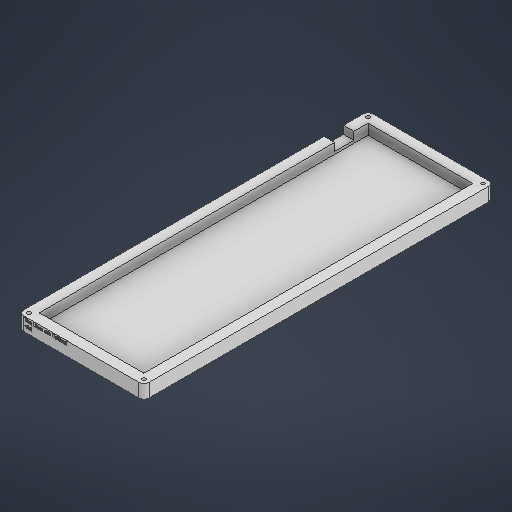
# Autodesk Inventor part: Bottom_Plate_MKey
Saved by Autodesk Inventor 2026 (Build 300175050, 175E)
## iProperties
Created: 2025-06-24
Part Number: Bottom_Plate_MKey
Material: Generic
Document SubType Name: Modeling
Designer: SaiAn
Density: 1 g/cm^3
Appearance: Default
Author: SaiAn
Autodesk Inventor part; units mm, degrees
ref_plane "YZ Plane" through (0, 0, 0) normal (1, 0, 0) x (0, 1, 0)
ref_plane "XZ Plane" through (0, 0, 0) normal (0, 1, 0) x (-1, 0, 0)
ref_plane "XY Plane" through (0, 0, 0) normal (0, 0, 1) x (1, 0, 0)
sketch "Sketch1" plane through (0, 0, 0) normal (0, 1, 0) x (-1, 0, 0)
  line L0 (0, 0) -> (100.47, 0)
  line L1 (100.47, 0) -> (100.47, -315.78)
  line L2 (100.47, -315.78) -> (0, -315.78)
  line L3 (0, -315.78) -> (0, 0)
  line L4 (110.47, 10) -> (-10, 10)
  line L5 (-10, 10) -> (-10, -325.78)
  line L6 (-10, -325.78) -> (110.47, -325.78)
  line L7 (110.47, -325.78) -> (110.47, 10)
  circle A0 centre (105.47, 5) radius 1.7
  circle A1 centre (-5, 5) radius 1.7
  circle A2 centre (-5, -320.78) radius 1.7
  circle A3 centre (105.47, -320.78) radius 1.7
  circle A4 centre (105.47, 5) radius 3
  circle A5 centre (-5, 5) radius 3
  circle A6 centre (-5, -320.78) radius 3
  circle A7 centre (105.47, -320.78) radius 3
  dimension "d0" = 100.47
  dimension "d1" = 315.78
  dimension "d2" = 120.47
  dimension "d3" = 335.78
  dimension "d4" = 10
  dimension "d5" = 10
  dimension "d6" = 3.4
  dimension "d7" = 3.4
  dimension "d8" = 3.4
  dimension "d9" = 3.4
  dimension "d10" = 5
  dimension "d11" = 5
  dimension "d12" = 5
  dimension "d13" = 5
  dimension "d14" = 5
  dimension "d15" = 5
  dimension "d16" = 5
  dimension "d17" = 5
  dimension "d18" = 6
  dimension "d19" = 6
  dimension "d20" = 6
  dimension "d21" = 6
  constraints: 16 end point, 8 centre point, 4 coincident, 4 parallel, 2 horizontal, 2 perpendicular
  measures "d0" distance of L1.end L2.end
  measures "d1" distance of L0.end L1.end
  measures "d2" distance of L6.end L5.end
  measures "d3" distance of L5.end L4.end
  measures "d4" distance between parallel lines of L1 L7
  measures "d5" distance between parallel lines of L6 L2
  measures "d6" diameter of A0
  measures "d7" diameter of A1
  measures "d8" diameter of A2
  measures "d9" diameter of A3
  measures "d10" distance from line of L7 A0.centre
  measures "d11" distance from line of L4 A0.centre
  measures "d12" distance from line of L5 A1.centre
  measures "d13" distance from line of L4 A1.centre
  measures "d14" distance from line of L5 A2.centre
  measures "d15" distance from line of L6 A2.centre
  measures "d16" distance from line of L7 A3.centre
  measures "d17" distance from line of L6 A3.centre
  measures "d18" diameter of A4
  measures "d19" diameter of A5
  measures "d20" diameter of A6
  measures "d21" diameter of A7
extrude "Extrusion1" add sketch "Sketch1" along normal blind 13 contours A4 | A5 | A6 | A7
extrude "Extrusion2" cut sketch "Sketch1" along normal blind 3.1 contours A4 | A5 | A6 | A7
extrude "Extrusion3" add sketch "Sketch1" along normal blind 13 contours L7 L6 L5 L4
extrude "Extrusion4" add sketch "Sketch1" along normal blind 3 contours L0 L1 L2 L3
sketch "Sketch3" plane through (0, 13, 0) normal (0, 1, 0) x (1, 0, 0)
  line L0 (-100.47, 0) -> (-100.47, 315.78) projected
  line L1 (-110.47, 325.78) -> (-110.47, -10) projected
  line L2 (-100.47, 302.18) -> (-110.47, 302.18)
  line L3 (-110.47, 302.18) -> (-110.47, 283.68)
  line L4 (-110.47, 283.68) -> (-100.47, 283.68)
  line L5 (-100.47, 283.68) -> (-100.47, 302.18)
  line L6 (10, 325.78) -> (-110.47, 325.78) projected
  point P0 (0, 0)
  dimension "d30" = 18.5
  dimension "d31" = 23.6
  constraints: 8 end point, 2 parallel, 2 point on line, 1 horizontal, 1 perpendicular
  measures "d30" distance of L3.end L2.end
  measures "d31" distance between parallel lines of L6 L2
extrude "Extrusion5" cut sketch "Sketch3" against normal blind 7.5
fillet "Fillet1" radius 5 3 edges at (-110.47, 6.5, -325.78) (10, 6.5, -325.78) (10, 6.5, 10)
fillet "Fillet2" radius 5 1 edges at (-110.47, 6.5, 10)
sketch "Sketch6" plane through (5, 0, 10) normal (0, 0, 1) x (1, 0, 0)
  line L0 (-109.6775, 12.2392) -> (-5.1074, 12.2392) construction
  line L1 (-5.1074, 12.2392) -> (-5.1074, 1.2883) construction
  line L2 (-5.1074, 1.2883) -> (-109.6775, 1.2883) construction
  line L3 (-109.6775, 1.2883) -> (-109.6775, 12.2392) construction
  line L4 (-108.6574, 9.0554) -> (-108.6574, 11.7427)
  line L5 (-108.6574, 11.7427) -> (-109.68, 11.7427)
  line L6 (-109.68, 11.7427) -> (-109.68, 12.1034)
  line L7 (-109.68, 12.1034) -> (-107.2297, 12.1034)
  line L8 (-107.2297, 12.1034) -> (-107.2297, 11.7427)
  line L9 (-107.2297, 11.7427) -> (-108.2523, 11.7427)
  line L10 (-108.2523, 11.7427) -> (-108.2523, 9.0554)
  line L11 (-108.2523, 9.0554) -> (-108.6574, 9.0554)
  line L12 (-105.1549, 9.0554) -> (-105.5402, 9.0554)
  line L13 (-105.5402, 9.0554) -> (-105.5402, 10.3595)
  spline S0 degree 2 poles (-105.5402, 10.3595) (-105.5402, 10.5176) (-105.5699, 10.7893) (-105.6143, 10.8708) knots 0 0 0 1 2 2 2
  spline S1 degree 2 poles (-105.6143, 10.8708) (-105.6612, 10.9573) (-105.8292, 11.0413) (-105.9725, 11.0413) knots 0 0 0 1 2 2 2
  spline S2 degree 2 poles (-105.9725, 11.0413) (-106.1157, 11.0413) (-106.4195, 10.8881) (-106.5653, 10.7646) knots 0 0 0 1 2 2 2
  line L14 (-106.5653, 10.7646) -> (-106.5653, 9.0554)
  line L15 (-106.5653, 9.0554) -> (-106.9506, 9.0554)
  line L16 (-106.9506, 9.0554) -> (-106.9506, 12.2392)
  line L17 (-106.9506, 12.2392) -> (-106.5653, 12.2392)
  line L18 (-106.5653, 12.2392) -> (-106.5653, 11.0882)
  spline S3 degree 2 poles (-106.5653, 11.0882) (-106.3924, 11.2438) (-106.0589, 11.4068) (-105.8712, 11.4068) knots 0 0 0 1 2 2 2
  spline S4 degree 2 poles (-105.8712, 11.4068) (-105.5353, 11.4068) (-105.1549, 10.9622) (-105.1549, 10.5398) knots 0 0 0 1 2 2 2
  line L19 (-105.1549, 10.5398) -> (-105.1549, 9.0554)
  spline S5 degree 2 poles (-103.621, 9.0035) (-104.1694, 9.0035) (-104.772, 9.6185) (-104.772, 10.1866) knots 0 0 0 1 2 2 2
  spline S6 degree 2 poles (-104.772, 10.1866) (-104.772, 10.7449) (-104.1867, 11.4068) (-103.7149, 11.4068) knots 0 0 0 1 2 2 2
  spline S7 degree 2 poles (-103.7149, 11.4068) (-103.5025, 11.4068) (-103.1739, 11.2833) (-103.0529, 11.1524) knots 0 0 0 1 2 2 2
  spline S8 degree 2 poles (-103.0529, 11.1524) (-102.9294, 11.0215) (-102.7985, 10.6436) (-102.7985, 10.3694) knots 0 0 0 1 2 2 2
  line L20 (-102.7985, 10.3694) -> (-102.7985, 10.1595)
  line L21 (-102.7985, 10.1595) -> (-104.3818, 10.1595)
  spline S9 degree 2 poles (-104.3818, 10.1595) (-104.3818, 9.7618) (-103.9816, 9.3394) (-103.626, 9.3394) knots 0 0 0 1 2 2 2
  spline S10 degree 2 poles (-103.626, 9.3394) (-103.5, 9.3394) (-103.2555, 9.3962) (-103.1567, 9.4407) knots 0 0 0 1 2 2 2
  spline S11 degree 2 poles (-103.1567, 9.4407) (-103.0529, 9.4901) (-102.9097, 9.5765) (-102.8627, 9.6161) knots 0 0 0 1 2 2 2
  line L22 (-102.8627, 9.6161) -> (-102.8405, 9.6161)
  line L23 (-102.8405, 9.6161) -> (-102.8405, 9.1962)
  spline S12 degree 2 poles (-102.8405, 9.1962) (-102.9072, 9.169) (-103.1097, 9.0899) (-103.1888, 9.0677) knots 0 0 0 1 2 2 2
  spline S13 degree 2 poles (-103.1888, 9.0677) (-103.2999, 9.0356) (-103.4827, 9.0035) (-103.621, 9.0035) knots 0 0 0 1 2 2 2
  spline S14 degree 2 poles (-103.1739, 10.4534) (-103.1789, 10.609) (-103.2431, 10.8362) (-103.3049, 10.9128) knots 0 0 0 1 2 2 2
  spline S15 degree 2 poles (-103.3049, 10.9128) (-103.3715, 10.9993) (-103.5815, 11.0907) (-103.7371, 11.0907) knots 0 0 0 1 2 2 2
  spline S16 degree 2 poles (-103.7371, 11.0907) (-103.8902, 11.0907) (-104.1051, 10.9993) (-104.1941, 10.9103) knots 0 0 0 1 2 2 2
  spline S17 degree 2 poles (-104.1941, 10.9103) (-104.2805, 10.819) (-104.3694, 10.5991) (-104.3818, 10.4534) knots 0 0 0 1 2 2 2
  line L24 (-104.3818, 10.4534) -> (-103.1739, 10.4534)
  line L25 (-99.3034, 9.0554) -> (-101.0695, 9.0554)
  line L26 (-101.0695, 9.0554) -> (-101.0695, 12.1034)
  line L27 (-101.0695, 12.1034) -> (-100.6644, 12.1034)
  line L28 (-100.6644, 12.1034) -> (-100.6644, 9.416)
  line L29 (-100.6644, 9.416) -> (-99.3034, 9.416)
  line L30 (-99.3034, 9.416) -> (-99.3034, 9.0554)
  line L31 (-98.6217, 9.0554) -> (-99.007, 9.0554)
  line L32 (-99.007, 9.0554) -> (-99.007, 11.3426)
  line L33 (-99.007, 11.3426) -> (-98.6217, 11.3426)
  line L34 (-98.6217, 11.3426) -> (-98.6217, 9.0554)
  line L35 (-98.5945, 11.723) -> (-99.0317, 11.723)
  line L36 (-99.0317, 11.723) -> (-99.0317, 12.1231)
  line L37 (-99.0317, 12.1231) -> (-98.5945, 12.1231)
  line L38 (-98.5945, 12.1231) -> (-98.5945, 11.723)
  line L39 (-96.2604, 9.0554) -> (-96.6457, 9.0554)
  line L40 (-96.6457, 9.0554) -> (-96.6457, 10.3595)
  spline S18 degree 2 poles (-96.6457, 10.3595) (-96.6457, 10.5176) (-96.6753, 10.7893) (-96.7198, 10.8708) knots 0 0 0 1 2 2 2
  spline S19 degree 2 poles (-96.7198, 10.8708) (-96.7667, 10.9573) (-96.9347, 11.0413) (-97.0779, 11.0413) knots 0 0 0 1 2 2 2
  spline S20 degree 2 poles (-97.0779, 11.0413) (-97.2212, 11.0413) (-97.525, 10.8881) (-97.6707, 10.7646) knots 0 0 0 1 2 2 2
  line L41 (-97.6707, 10.7646) -> (-97.6707, 9.0554)
  line L42 (-97.6707, 9.0554) -> (-98.0561, 9.0554)
  line L43 (-98.0561, 9.0554) -> (-98.0561, 11.3426)
  line L44 (-98.0561, 11.3426) -> (-97.6707, 11.3426)
  line L45 (-97.6707, 11.3426) -> (-97.6707, 11.0882)
  spline S21 degree 2 poles (-97.6707, 11.0882) (-97.4978, 11.2438) (-97.1644, 11.4068) (-96.9767, 11.4068) knots 0 0 0 1 2 2 2
  spline S22 degree 2 poles (-96.9767, 11.4068) (-96.6408, 11.4068) (-96.2604, 10.9622) (-96.2604, 10.5398) knots 0 0 0 1 2 2 2
  line L46 (-96.2604, 10.5398) -> (-96.2604, 9.0554)
  spline S23 degree 2 poles (-94.7265, 9.0035) (-95.2748, 9.0035) (-95.8775, 9.6185) (-95.8775, 10.1866) knots 0 0 0 1 2 2 2
  spline S24 degree 2 poles (-95.8775, 10.1866) (-95.8775, 10.7449) (-95.2921, 11.4068) (-94.8203, 11.4068) knots 0 0 0 1 2 2 2
  spline S25 degree 2 poles (-94.8203, 11.4068) (-94.6079, 11.4068) (-94.2794, 11.2833) (-94.1584, 11.1524) knots 0 0 0 1 2 2 2
  spline S26 degree 2 poles (-94.1584, 11.1524) (-94.0349, 11.0215) (-93.904, 10.6436) (-93.904, 10.3694) knots 0 0 0 1 2 2 2
  line L47 (-93.904, 10.3694) -> (-93.904, 10.1595)
  line L48 (-93.904, 10.1595) -> (-95.4873, 10.1595)
  spline S27 degree 2 poles (-95.4873, 10.1595) (-95.4873, 9.7618) (-95.0871, 9.3394) (-94.7314, 9.3394) knots 0 0 0 1 2 2 2
  spline S28 degree 2 poles (-94.7314, 9.3394) (-94.6055, 9.3394) (-94.3609, 9.3962) (-94.2621, 9.4407) knots 0 0 0 1 2 2 2
  spline S29 degree 2 poles (-94.2621, 9.4407) (-94.1584, 9.4901) (-94.0151, 9.5765) (-93.9682, 9.6161) knots 0 0 0 1 2 2 2
  line L49 (-93.9682, 9.6161) -> (-93.946, 9.6161)
  line L50 (-93.946, 9.6161) -> (-93.946, 9.1962)
  spline S30 degree 2 poles (-93.946, 9.1962) (-94.0127, 9.169) (-94.2152, 9.0899) (-94.2942, 9.0677) knots 0 0 0 1 2 2 2
  spline S31 degree 2 poles (-94.2942, 9.0677) (-94.4054, 9.0356) (-94.5882, 9.0035) (-94.7265, 9.0035) knots 0 0 0 1 2 2 2
  spline S32 degree 2 poles (-94.2794, 10.4534) (-94.2844, 10.609) (-94.3486, 10.8362) (-94.4103, 10.9128) knots 0 0 0 1 2 2 2
  spline S33 degree 2 poles (-94.4103, 10.9128) (-94.477, 10.9993) (-94.687, 11.0907) (-94.8426, 11.0907) knots 0 0 0 1 2 2 2
  spline S34 degree 2 poles (-94.8426, 11.0907) (-94.9957, 11.0907) (-95.2106, 10.9993) (-95.2995, 10.9103) knots 0 0 0 1 2 2 2
  spline S35 degree 2 poles (-95.2995, 10.9103) (-95.386, 10.819) (-95.4749, 10.5991) (-95.4873, 10.4534) knots 0 0 0 1 2 2 2
  line L51 (-95.4873, 10.4534) -> (-94.2794, 10.4534)
  spline S36 degree 2 poles (-92.8962, 9.001) (-93.1259, 9.001) (-93.5236, 9.1245) (-93.6545, 9.1937) knots 0 0 0 1 2 2 2
  line L52 (-93.6545, 9.1937) -> (-93.6545, 9.6259)
  line L53 (-93.6545, 9.6259) -> (-93.6347, 9.6259)
  spline S37 degree 2 poles (-93.6347, 9.6259) (-93.5853, 9.5864) (-93.452, 9.4926) (-93.3408, 9.4407) knots 0 0 0 1 2 2 2
  spline S38 degree 2 poles (-93.3408, 9.4407) (-93.2445, 9.3938) (-93.0074, 9.3246) (-92.8814, 9.3246) knots 0 0 0 1 2 2 2
  spline S39 degree 2 poles (-92.8814, 9.3246) (-92.79, 9.3246) (-92.58, 9.3666) (-92.5306, 9.4012) knots 0 0 0 1 2 2 2
  spline S40 degree 2 poles (-92.5306, 9.4012) (-92.459, 9.4481) (-92.3948, 9.5543) (-92.3948, 9.663) knots 0 0 0 1 2 2 2
  spline S41 degree 2 poles (-92.3948, 9.663) (-92.3948, 9.7988) (-92.543, 9.9396) (-92.7332, 9.9866) knots 0 0 0 1 2 2 2
  spline S42 degree 2 poles (-92.7332, 9.9866) (-92.8073, 10.0039) (-93.0444, 10.0533) (-93.1457, 10.0804) knots 0 0 0 1 2 2 2
  spline S43 degree 2 poles (-93.1457, 10.0804) (-93.4075, 10.157) (-93.6446, 10.4732) (-93.6446, 10.6979) knots 0 0 0 1 2 2 2
  spline S44 degree 2 poles (-93.6446, 10.6979) (-93.6446, 11.0091) (-93.1778, 11.3969) (-92.7925, 11.3969) knots 0 0 0 1 2 2 2
  spline S45 degree 2 poles (-92.7925, 11.3969) (-92.6023, 11.3969) (-92.217, 11.3031) (-92.086, 11.2314) knots 0 0 0 1 2 2 2
  line L54 (-92.086, 11.2314) -> (-92.086, 10.819)
  line L55 (-92.086, 10.819) -> (-92.1058, 10.819)
  spline S46 degree 2 poles (-92.1058, 10.819) (-92.254, 10.9375) (-92.6146, 11.0734) (-92.7999, 11.0734) knots 0 0 0 1 2 2 2
  spline S47 degree 2 poles (-92.7999, 11.0734) (-92.9901, 11.0734) (-93.2519, 10.9128) (-93.2519, 10.7523) knots 0 0 0 1 2 2 2
  spline S48 degree 2 poles (-93.2519, 10.7523) (-93.2519, 10.6065) (-93.0963, 10.4657) (-92.9234, 10.4213) knots 0 0 0 1 2 2 2
  spline S49 degree 2 poles (-92.9234, 10.4213) (-92.8394, 10.3991) (-92.627, 10.3546) (-92.5109, 10.3274) knots 0 0 0 1 2 2 2
  spline S50 degree 2 poles (-92.5109, 10.3274) (-92.2589, 10.2632) (-92.0021, 9.9693) (-92.0021, 9.7149) knots 0 0 0 1 2 2 2
  spline S51 degree 2 poles (-92.0021, 9.7149) (-92.0021, 9.5667) (-92.1182, 9.3048) (-92.2318, 9.2085) knots 0 0 0 1 2 2 2
  spline S52 degree 2 poles (-92.2318, 9.2085) (-92.3528, 9.1072) (-92.6616, 9.001) (-92.8962, 9.001) knots 0 0 0 1 2 2 2
  spline S53 degree 2 poles (-89.0603, 9.2974) (-89.1072, 9.2628) (-89.2653, 9.1393) (-89.3394, 9.1023) knots 0 0 0 1 2 2 2
  spline S54 degree 2 poles (-89.3394, 9.1023) (-89.4407, 9.048) (-89.6308, 8.9911) (-89.8037, 8.9911) knots 0 0 0 1 2 2 2
  spline S55 degree 2 poles (-89.8037, 8.9911) (-89.9445, 8.9911) (-90.1989, 9.0974) (-90.2953, 9.1937) knots 0 0 0 1 2 2 2
  spline S56 degree 2 poles (-90.2953, 9.1937) (-90.3867, 9.2875) (-90.4978, 9.5642) (-90.4978, 9.7173) knots 0 0 0 1 2 2 2
  spline S57 degree 2 poles (-90.4978, 9.7173) (-90.4978, 9.9544) (-90.2977, 10.2904) (-90.0804, 10.3867) knots 0 0 0 1 2 2 2
  spline S58 degree 2 poles (-90.0804, 10.3867) (-89.8877, 10.4756) (-89.3641, 10.5423) (-89.0603, 10.5596) knots 0 0 0 1 2 2 2
  line L56 (-89.0603, 10.5596) -> (-89.0603, 10.6337)
  spline S59 degree 2 poles (-89.0603, 10.6337) (-89.0603, 10.7671) (-89.1418, 10.9326) (-89.2159, 10.9795) knots 0 0 0 1 2 2 2
  spline S60 degree 2 poles (-89.2159, 10.9795) (-89.29, 11.0264) (-89.5024, 11.0561) (-89.616, 11.0561) knots 0 0 0 1 2 2 2
  spline S61 degree 2 poles (-89.616, 11.0561) (-89.7494, 11.0561) (-90.11, 10.977) (-90.2903, 10.9005) knots 0 0 0 1 2 2 2
  line L57 (-90.2903, 10.9005) -> (-90.3126, 10.9005)
  line L58 (-90.3126, 10.9005) -> (-90.3126, 11.2932)
  spline S62 degree 2 poles (-90.3126, 11.2932) (-90.2064, 11.3228) (-89.8087, 11.3969) (-89.6136, 11.3969) knots 0 0 0 1 2 2 2
  spline S63 degree 2 poles (-89.6136, 11.3969) (-89.3764, 11.3969) (-89.0529, 11.3228) (-88.9244, 11.2265) knots 0 0 0 1 2 2 2
  spline S64 degree 2 poles (-88.9244, 11.2265) (-88.7984, 11.1326) (-88.6749, 10.8338) (-88.6749, 10.6189) knots 0 0 0 1 2 2 2
  line L59 (-88.6749, 10.6189) -> (-88.6749, 9.0554)
  line L60 (-88.6749, 9.0554) -> (-89.0603, 9.0554)
  line L61 (-89.0603, 9.0554) -> (-89.0603, 9.2974)
  line L62 (-89.0603, 9.6185) -> (-89.0603, 10.2533)
  spline S65 degree 2 poles (-89.0603, 10.2533) (-89.1986, 10.241) (-89.616, 10.199) (-89.7469, 10.1595) knots 0 0 0 1 2 2 2
  spline S66 degree 2 poles (-89.7469, 10.1595) (-89.9001, 10.1125) (-90.1001, 9.9174) (-90.1001, 9.7445) knots 0 0 0 1 2 2 2
  spline S67 degree 2 poles (-90.1001, 9.7445) (-90.1001, 9.5469) (-89.8778, 9.3468) (-89.6654, 9.3468) knots 0 0 0 1 2 2 2
  spline S68 degree 2 poles (-89.6654, 9.3468) (-89.4851, 9.3468) (-89.1887, 9.5024) (-89.0603, 9.6185) knots 0 0 0 1 2 2 2
  line L63 (-86.9212, 10.9301) -> (-86.941, 10.9301)
  spline S69 degree 2 poles (-86.941, 10.9301) (-86.9855, 10.9425) (-87.0818, 10.9474) (-87.1485, 10.9474) knots 0 0 0 1 2 2 2
  spline S70 degree 2 poles (-87.1485, 10.9474) (-87.3041, 10.9474) (-87.6104, 10.8115) (-87.7487, 10.6782) knots 0 0 0 1 2 2 2
  line L64 (-87.7487, 10.6782) -> (-87.7487, 9.0554)
  line L65 (-87.7487, 9.0554) -> (-88.134, 9.0554)
  line L66 (-88.134, 9.0554) -> (-88.134, 11.3426)
  line L67 (-88.134, 11.3426) -> (-87.7487, 11.3426)
  line L68 (-87.7487, 11.3426) -> (-87.7487, 11.0017)
  spline S71 degree 2 poles (-87.7487, 11.0017) (-87.5387, 11.1895) (-87.225, 11.3426) (-87.0768, 11.3426) knots 0 0 0 1 2 2 2
  spline S72 degree 2 poles (-87.0768, 11.3426) (-87.0176, 11.3426) (-86.9583, 11.3377) (-86.9212, 11.3302) knots 0 0 0 1 2 2 2
  line L69 (-86.9212, 11.3302) -> (-86.9212, 10.9301)
  spline S73 degree 2 poles (-85.6294, 9.0035) (-86.1778, 9.0035) (-86.7804, 9.6185) (-86.7804, 10.1866) knots 0 0 0 1 2 2 2
  spline S74 degree 2 poles (-86.7804, 10.1866) (-86.7804, 10.7449) (-86.1951, 11.4068) (-85.7233, 11.4068) knots 0 0 0 1 2 2 2
  spline S75 degree 2 poles (-85.7233, 11.4068) (-85.5109, 11.4068) (-85.1823, 11.2833) (-85.0613, 11.1524) knots 0 0 0 1 2 2 2
  spline S76 degree 2 poles (-85.0613, 11.1524) (-84.9378, 11.0215) (-84.8069, 10.6436) (-84.8069, 10.3694) knots 0 0 0 1 2 2 2
  line L70 (-84.8069, 10.3694) -> (-84.8069, 10.1595)
  line L71 (-84.8069, 10.1595) -> (-86.3902, 10.1595)
  spline S77 degree 2 poles (-86.3902, 10.1595) (-86.3902, 9.7618) (-85.99, 9.3394) (-85.6344, 9.3394) knots 0 0 0 1 2 2 2
  spline S78 degree 2 poles (-85.6344, 9.3394) (-85.5084, 9.3394) (-85.2639, 9.3962) (-85.1651, 9.4407) knots 0 0 0 1 2 2 2
  spline S79 degree 2 poles (-85.1651, 9.4407) (-85.0613, 9.4901) (-84.9181, 9.5765) (-84.8711, 9.6161) knots 0 0 0 1 2 2 2
  line L72 (-84.8711, 9.6161) -> (-84.8489, 9.6161)
  line L73 (-84.8489, 9.6161) -> (-84.8489, 9.1962)
  spline S80 degree 2 poles (-84.8489, 9.1962) (-84.9156, 9.169) (-85.1181, 9.0899) (-85.1972, 9.0677) knots 0 0 0 1 2 2 2
  spline S81 degree 2 poles (-85.1972, 9.0677) (-85.3083, 9.0356) (-85.4911, 9.0035) (-85.6294, 9.0035) knots 0 0 0 1 2 2 2
  spline S82 degree 2 poles (-85.1823, 10.4534) (-85.1873, 10.609) (-85.2515, 10.8362) (-85.3133, 10.9128) knots 0 0 0 1 2 2 2
  spline S83 degree 2 poles (-85.3133, 10.9128) (-85.3799, 10.9993) (-85.5899, 11.0907) (-85.7455, 11.0907) knots 0 0 0 1 2 2 2
  spline S84 degree 2 poles (-85.7455, 11.0907) (-85.8986, 11.0907) (-86.1135, 10.9993) (-86.2025, 10.9103) knots 0 0 0 1 2 2 2
  spline S85 degree 2 poles (-86.2025, 10.9103) (-86.2889, 10.819) (-86.3778, 10.5991) (-86.3902, 10.4534) knots 0 0 0 1 2 2 2
  line L74 (-86.3902, 10.4534) -> (-85.1823, 10.4534)
  spline S86 degree 2 poles (-80.9216, 11.7551) (-80.7487, 11.5526) (-80.556, 10.9597) (-80.556, 10.5794) knots 0 0 0 1 2 2 2
  spline S87 degree 2 poles (-80.556, 10.5794) (-80.556, 10.2089) (-80.7437, 9.6086) (-80.9216, 9.4061) knots 0 0 0 1 2 2 2
  spline S88 degree 2 poles (-80.9216, 9.4061) (-81.1093, 9.1937) (-81.6058, 8.9911) (-81.9046, 8.9911) knots 0 0 0 1 2 2 2
  spline S89 degree 2 poles (-81.9046, 8.9911) (-82.2134, 8.9911) (-82.7074, 9.2011) (-82.8877, 9.4061) knots 0 0 0 1 2 2 2
  spline S90 degree 2 poles (-82.8877, 9.4061) (-83.0631, 9.6086) (-83.2508, 10.2039) (-83.2508, 10.5794) knots 0 0 0 1 2 2 2
  spline S91 degree 2 poles (-83.2508, 10.5794) (-83.2508, 10.9622) (-83.0606, 11.5451) (-82.8852, 11.7551) knots 0 0 0 1 2 2 2
  spline S92 degree 2 poles (-82.8852, 11.7551) (-82.7074, 11.9576) (-82.2109, 12.1676) (-81.9046, 12.1676) knots 0 0 0 1 2 2 2
  spline S93 degree 2 poles (-81.9046, 12.1676) (-81.5934, 12.1676) (-81.0945, 11.9502) (-80.9216, 11.7551) knots 0 0 0 1 2 2 2
  spline S94 degree 2 poles (-80.9784, 10.5794) (-80.9784, 10.8807) (-81.1093, 11.3475) (-81.2278, 11.5007) knots 0 0 0 1 2 2 2
  spline S95 degree 2 poles (-81.2278, 11.5007) (-81.3489, 11.6588) (-81.6897, 11.8168) (-81.9022, 11.8168) knots 0 0 0 1 2 2 2
  spline S96 degree 2 poles (-81.9022, 11.8168) (-82.122, 11.8168) (-82.453, 11.6637) (-82.5789, 11.5007) knots 0 0 0 1 2 2 2
  spline S97 degree 2 poles (-82.5789, 11.5007) (-82.7, 11.3451) (-82.8284, 10.8758) (-82.8284, 10.5794) knots 0 0 0 1 2 2 2
  spline S98 degree 2 poles (-82.8284, 10.5794) (-82.8284, 9.9791) (-82.3245, 9.3419) (-81.9022, 9.3419) knots 0 0 0 1 2 2 2
  spline S99 degree 2 poles (-81.9022, 9.3419) (-81.4798, 9.3419) (-80.9784, 9.9791) (-80.9784, 10.5794) knots 0 0 0 1 2 2 2
  spline S100 degree 2 poles (-78.2243, 10.2607) (-78.2243, 9.6877) (-78.7702, 9.0109) (-79.1876, 9.0109) knots 0 0 0 1 2 2 2
  spline S101 degree 2 poles (-79.1876, 9.0109) (-79.358, 9.0109) (-79.6199, 9.0899) (-79.7557, 9.1715) knots 0 0 0 1 2 2 2
  line L75 (-79.7557, 9.1715) -> (-79.7557, 8.2131)
  line L76 (-79.7557, 8.2131) -> (-80.141, 8.2131)
  line L77 (-80.141, 8.2131) -> (-80.141, 11.3426)
  line L78 (-80.141, 11.3426) -> (-79.7557, 11.3426)
  line L79 (-79.7557, 11.3426) -> (-79.7557, 11.103)
  spline S102 degree 2 poles (-79.7557, 11.103) (-79.6125, 11.2339) (-79.2617, 11.4068) (-79.0567, 11.4068) knots 0 0 0 1 2 2 2
  spline S103 degree 2 poles (-79.0567, 11.4068) (-78.664, 11.4068) (-78.2243, 10.7844) (-78.2243, 10.2607) knots 0 0 0 1 2 2 2
  spline S104 degree 2 poles (-78.622, 10.2163) (-78.622, 10.609) (-78.8715, 11.0413) (-79.1506, 11.0413) knots 0 0 0 1 2 2 2
  spline S105 degree 2 poles (-79.1506, 11.0413) (-79.3136, 11.0413) (-79.6199, 10.8955) (-79.7557, 10.7819) knots 0 0 0 1 2 2 2
  line L80 (-79.7557, 10.7819) -> (-79.7557, 9.4827)
  spline S106 degree 2 poles (-79.7557, 9.4827) (-79.605, 9.411) (-79.3902, 9.3567) (-79.2518, 9.3567) knots 0 0 0 1 2 2 2
  spline S107 degree 2 poles (-79.2518, 9.3567) (-78.953, 9.3567) (-78.622, 9.7964) (-78.622, 10.2163) knots 0 0 0 1 2 2 2
  spline S108 degree 2 poles (-77.1326, 9.0109) (-77.4463, 9.0109) (-77.7995, 9.3691) (-77.7995, 9.7568) knots 0 0 0 1 2 2 2
  line L81 (-77.7995, 9.7568) -> (-77.7995, 11.024)
  line L82 (-77.7995, 11.024) -> (-78.0588, 11.024)
  line L83 (-78.0588, 11.024) -> (-78.0588, 11.3426)
  line L84 (-78.0588, 11.3426) -> (-77.7995, 11.3426)
  line L85 (-77.7995, 11.3426) -> (-77.7995, 11.9996)
  line L86 (-77.7995, 11.9996) -> (-77.4141, 11.9996)
  line L87 (-77.4141, 11.9996) -> (-77.4141, 11.3426)
  line L88 (-77.4141, 11.3426) -> (-76.7052, 11.3426)
  line L89 (-76.7052, 11.3426) -> (-76.7052, 11.024)
  line L90 (-76.7052, 11.024) -> (-77.4141, 11.024)
  line L91 (-77.4141, 11.024) -> (-77.4141, 9.9347)
  spline S109 degree 2 poles (-77.4141, 9.9347) (-77.4141, 9.7618) (-77.4018, 9.5716) (-77.3598, 9.4901) knots 0 0 0 1 2 2 2
  spline S110 degree 2 poles (-77.3598, 9.4901) (-77.3252, 9.4185) (-77.1696, 9.3468) (-77.0362, 9.3468) knots 0 0 0 1 2 2 2
  spline S111 degree 2 poles (-77.0362, 9.3468) (-76.9424, 9.3468) (-76.767, 9.4036) (-76.7275, 9.4209) knots 0 0 0 1 2 2 2
  line L92 (-76.7275, 9.4209) -> (-76.7052, 9.4209)
  line L93 (-76.7052, 9.4209) -> (-76.7052, 9.0751)
  spline S112 degree 2 poles (-76.7052, 9.0751) (-76.8139, 9.0455) (-77.0362, 9.0109) (-77.1326, 9.0109) knots 0 0 0 1 2 2 2
  line L94 (-76.0285, 9.0554) -> (-76.4138, 9.0554)
  line L95 (-76.4138, 9.0554) -> (-76.4138, 11.3426)
  line L96 (-76.4138, 11.3426) -> (-76.0285, 11.3426)
  line L97 (-76.0285, 11.3426) -> (-76.0285, 9.0554)
  line L98 (-76.0013, 11.723) -> (-76.4385, 11.723)
  line L99 (-76.4385, 11.723) -> (-76.4385, 12.1231)
  line L100 (-76.4385, 12.1231) -> (-76.0013, 12.1231)
  line L101 (-76.0013, 12.1231) -> (-76.0013, 11.723)
  line L102 (-72.8693, 9.0554) -> (-72.8693, 10.3793)
  spline S113 degree 2 poles (-72.8693, 10.3793) (-72.8693, 10.5374) (-72.894, 10.8066) (-72.9335, 10.8807) knots 0 0 0 1 2 2 2
  spline S114 degree 2 poles (-72.9335, 10.8807) (-72.9731, 10.9622) (-73.1237, 11.0413) (-73.2546, 11.0413) knots 0 0 0 1 2 2 2
  spline S115 degree 2 poles (-73.2546, 11.0413) (-73.3732, 11.0413) (-73.6449, 10.8955) (-73.7882, 10.7572) knots 0 0 0 1 2 2 2
  spline S116 degree 2 poles (-73.7882, 10.7572) (-73.7857, 10.7226) (-73.7808, 10.6263) (-73.7808, 10.5621) knots 0 0 0 1 2 2 2
  line L103 (-73.7808, 10.5621) -> (-73.7808, 9.0554)
  line L104 (-73.7808, 9.0554) -> (-74.1661, 9.0554)
  line L105 (-74.1661, 9.0554) -> (-74.1661, 10.3793)
  spline S117 degree 2 poles (-74.1661, 10.3793) (-74.1661, 10.5374) (-74.1908, 10.8066) (-74.2303, 10.8807) knots 0 0 0 1 2 2 2
  spline S118 degree 2 poles (-74.2303, 10.8807) (-74.2698, 10.9622) (-74.4205, 11.0413) (-74.5514, 11.0413) knots 0 0 0 1 2 2 2
  spline S119 degree 2 poles (-74.5514, 11.0413) (-74.6749, 11.0413) (-74.9491, 10.8856) (-75.0775, 10.7646) knots 0 0 0 1 2 2 2
  line L106 (-75.0775, 10.7646) -> (-75.0775, 9.0554)
  line L107 (-75.0775, 9.0554) -> (-75.4628, 9.0554)
  line L108 (-75.4628, 9.0554) -> (-75.4628, 11.3426)
  line L109 (-75.4628, 11.3426) -> (-75.0775, 11.3426)
  line L110 (-75.0775, 11.3426) -> (-75.0775, 11.0907)
  spline S120 degree 2 poles (-75.0775, 11.0907) (-74.9268, 11.2413) (-74.6304, 11.4068) (-74.4526, 11.4068) knots 0 0 0 1 2 2 2
  spline S121 degree 2 poles (-74.4526, 11.4068) (-74.2501, 11.4068) (-73.9364, 11.2216) (-73.8549, 11.0116) knots 0 0 0 1 2 2 2
  spline S122 degree 2 poles (-73.8549, 11.0116) (-73.6795, 11.2067) (-73.3485, 11.4068) (-73.1558, 11.4068) knots 0 0 0 1 2 2 2
  spline S123 degree 2 poles (-73.1558, 11.4068) (-73.0076, 11.4068) (-72.7656, 11.3154) (-72.6767, 11.2117) knots 0 0 0 1 2 2 2
  spline S124 degree 2 poles (-72.6767, 11.2117) (-72.5853, 11.1079) (-72.484, 10.7967) (-72.484, 10.5621) knots 0 0 0 1 2 2 2
  line L111 (-72.484, 10.5621) -> (-72.484, 9.0554)
  line L112 (-72.484, 9.0554) -> (-72.8693, 9.0554)
  spline S125 degree 2 poles (-70.6685, 9.2974) (-70.7155, 9.2628) (-70.8735, 9.1393) (-70.9476, 9.1023) knots 0 0 0 1 2 2 2
  spline S126 degree 2 poles (-70.9476, 9.1023) (-71.0489, 9.048) (-71.2391, 8.9911) (-71.412, 8.9911) knots 0 0 0 1 2 2 2
  spline S127 degree 2 poles (-71.412, 8.9911) (-71.5528, 8.9911) (-71.8072, 9.0974) (-71.9035, 9.1937) knots 0 0 0 1 2 2 2
  spline S128 degree 2 poles (-71.9035, 9.1937) (-71.9949, 9.2875) (-72.1061, 9.5642) (-72.1061, 9.7173) knots 0 0 0 1 2 2 2
  spline S129 degree 2 poles (-72.1061, 9.7173) (-72.1061, 9.9544) (-71.906, 10.2904) (-71.6886, 10.3867) knots 0 0 0 1 2 2 2
  spline S130 degree 2 poles (-71.6886, 10.3867) (-71.496, 10.4756) (-70.9723, 10.5423) (-70.6685, 10.5596) knots 0 0 0 1 2 2 2
  line L113 (-70.6685, 10.5596) -> (-70.6685, 10.6337)
  spline S131 degree 2 poles (-70.6685, 10.6337) (-70.6685, 10.7671) (-70.75, 10.9326) (-70.8241, 10.9795) knots 0 0 0 1 2 2 2
  spline S132 degree 2 poles (-70.8241, 10.9795) (-70.8982, 11.0264) (-71.1107, 11.0561) (-71.2243, 11.0561) knots 0 0 0 1 2 2 2
  spline S133 degree 2 poles (-71.2243, 11.0561) (-71.3577, 11.0561) (-71.7183, 10.977) (-71.8986, 10.9005) knots 0 0 0 1 2 2 2
  line L114 (-71.8986, 10.9005) -> (-71.9208, 10.9005)
  line L115 (-71.9208, 10.9005) -> (-71.9208, 11.2932)
  spline S134 degree 2 poles (-71.9208, 11.2932) (-71.8146, 11.3228) (-71.4169, 11.3969) (-71.2218, 11.3969) knots 0 0 0 1 2 2 2
  spline S135 degree 2 poles (-71.2218, 11.3969) (-70.9847, 11.3969) (-70.6611, 11.3228) (-70.5327, 11.2265) knots 0 0 0 1 2 2 2
  spline S136 degree 2 poles (-70.5327, 11.2265) (-70.4067, 11.1326) (-70.2832, 10.8338) (-70.2832, 10.6189) knots 0 0 0 1 2 2 2
  line L116 (-70.2832, 10.6189) -> (-70.2832, 9.0554)
  line L117 (-70.2832, 9.0554) -> (-70.6685, 9.0554)
  line L118 (-70.6685, 9.0554) -> (-70.6685, 9.2974)
  line L119 (-70.6685, 9.6185) -> (-70.6685, 10.2533)
  spline S137 degree 2 poles (-70.6685, 10.2533) (-70.8069, 10.241) (-71.2243, 10.199) (-71.3552, 10.1595) knots 0 0 0 1 2 2 2
  spline S138 degree 2 poles (-71.3552, 10.1595) (-71.5083, 10.1125) (-71.7084, 9.9174) (-71.7084, 9.7445) knots 0 0 0 1 2 2 2
  spline S139 degree 2 poles (-71.7084, 9.7445) (-71.7084, 9.5469) (-71.4861, 9.3468) (-71.2737, 9.3468) knots 0 0 0 1 2 2 2
  spline S140 degree 2 poles (-71.2737, 9.3468) (-71.0934, 9.3468) (-70.797, 9.5024) (-70.6685, 9.6185) knots 0 0 0 1 2 2 2
  line L120 (-69.3495, 9.0554) -> (-69.7349, 9.0554)
  line L121 (-69.7349, 9.0554) -> (-69.7349, 12.2392)
  line L122 (-69.7349, 12.2392) -> (-69.3495, 12.2392)
  line L123 (-69.3495, 12.2392) -> (-69.3495, 9.0554)
  line L124 (-108.3387, 5.1855) -> (-109.4922, 5.1855)
  line L125 (-109.4922, 5.1855) -> (-109.4922, 5.556)
  line L126 (-109.4922, 5.556) -> (-108.3387, 5.556)
  line L127 (-108.3387, 5.556) -> (-108.3387, 5.1855)
  spline S141 degree 2 poles (-106.9975, 3.9826) (-107.3285, 3.9826) (-107.7929, 4.1209) (-107.9979, 4.2197) knots 0 0 0 1 2 2 2
  line L128 (-107.9979, 4.2197) -> (-107.9979, 4.7285)
  line L129 (-107.9979, 4.7285) -> (-107.9682, 4.7285)
  spline S142 degree 2 poles (-107.9682, 4.7285) (-107.7682, 4.5408) (-107.2618, 4.3333) (-107.0272, 4.3333) knots 0 0 0 1 2 2 2
  spline S143 degree 2 poles (-107.0272, 4.3333) (-106.6912, 4.3333) (-106.3479, 4.6124) (-106.3479, 4.8421) knots 0 0 0 1 2 2 2
  spline S144 degree 2 poles (-106.3479, 4.8421) (-106.3479, 5.0249) (-106.5282, 5.2522) (-106.7234, 5.309) knots 0 0 0 1 2 2 2
  spline S145 degree 2 poles (-106.7234, 5.309) (-106.8641, 5.3485) (-107.0988, 5.4028) (-107.2742, 5.4473) knots 0 0 0 1 2 2 2
  spline S146 degree 2 poles (-107.2742, 5.4473) (-107.4323, 5.4893) (-107.6817, 5.6153) (-107.7781, 5.7165) knots 0 0 0 1 2 2 2
  spline S147 degree 2 poles (-107.7781, 5.7165) (-107.8719, 5.8178) (-107.9757, 6.0895) (-107.9757, 6.2673) knots 0 0 0 1 2 2 2
  spline S148 degree 2 poles (-107.9757, 6.2673) (-107.9757, 6.6378) (-107.3977, 7.1393) (-106.9506, 7.1393) knots 0 0 0 1 2 2 2
  spline S149 degree 2 poles (-106.9506, 7.1393) (-106.6937, 7.1393) (-106.2392, 7.038) (-106.0441, 6.9417) knots 0 0 0 1 2 2 2
  line L130 (-106.0441, 6.9417) -> (-106.0441, 6.4575)
  line L131 (-106.0441, 6.4575) -> (-106.0737, 6.4575)
  spline S150 degree 2 poles (-106.0737, 6.4575) (-106.2195, 6.5909) (-106.674, 6.7885) (-106.9234, 6.7885) knots 0 0 0 1 2 2 2
  spline S151 degree 2 poles (-106.9234, 6.7885) (-107.205, 6.7885) (-107.5533, 6.5242) (-107.5533, 6.3093) knots 0 0 0 1 2 2 2
  spline S152 degree 2 poles (-107.5533, 6.3093) (-107.5533, 6.1167) (-107.3483, 5.887) (-107.1556, 5.8351) knots 0 0 0 1 2 2 2
  spline S153 degree 2 poles (-107.1556, 5.8351) (-107.0272, 5.8005) (-106.6542, 5.7116) (-106.5307, 5.6745) knots 0 0 0 1 2 2 2
  spline S154 degree 2 poles (-106.5307, 5.6745) (-106.217, 5.5782) (-105.9255, 5.1904) (-105.9255, 4.9064) knots 0 0 0 1 2 2 2
  spline S155 degree 2 poles (-105.9255, 4.9064) (-105.9255, 4.726) (-106.0713, 4.3802) (-106.2022, 4.2592) knots 0 0 0 1 2 2 2
  spline S156 degree 2 poles (-106.2022, 4.2592) (-106.3479, 4.1258) (-106.7184, 3.9826) (-106.9975, 3.9826) knots 0 0 0 1 2 2 2
  spline S157 degree 2 poles (-104.2682, 4.279) (-104.3151, 4.2444) (-104.4732, 4.1209) (-104.5473, 4.0838) knots 0 0 0 1 2 2 2
  spline S158 degree 2 poles (-104.5473, 4.0838) (-104.6485, 4.0295) (-104.8387, 3.9727) (-105.0116, 3.9727) knots 0 0 0 1 2 2 2
  spline S159 degree 2 poles (-105.0116, 3.9727) (-105.1524, 3.9727) (-105.4068, 4.0789) (-105.5032, 4.1752) knots 0 0 0 1 2 2 2
  spline S160 degree 2 poles (-105.5032, 4.1752) (-105.5946, 4.2691) (-105.7057, 4.5457) (-105.7057, 4.6989) knots 0 0 0 1 2 2 2
  spline S161 degree 2 poles (-105.7057, 4.6989) (-105.7057, 4.936) (-105.5056, 5.2719) (-105.2883, 5.3683) knots 0 0 0 1 2 2 2
  spline S162 degree 2 poles (-105.2883, 5.3683) (-105.0956, 5.4572) (-104.572, 5.5239) (-104.2682, 5.5412) knots 0 0 0 1 2 2 2
  line L132 (-104.2682, 5.5412) -> (-104.2682, 5.6153)
  spline S163 degree 2 poles (-104.2682, 5.6153) (-104.2682, 5.7486) (-104.3497, 5.9141) (-104.4238, 5.9611) knots 0 0 0 1 2 2 2
  spline S164 degree 2 poles (-104.4238, 5.9611) (-104.4979, 6.008) (-104.7103, 6.0376) (-104.8239, 6.0376) knots 0 0 0 1 2 2 2
  spline S165 degree 2 poles (-104.8239, 6.0376) (-104.9573, 6.0376) (-105.3179, 5.9586) (-105.4982, 5.882) knots 0 0 0 1 2 2 2
  line L133 (-105.4982, 5.882) -> (-105.5205, 5.882)
  line L134 (-105.5205, 5.882) -> (-105.5205, 6.2747)
  spline S166 degree 2 poles (-105.5205, 6.2747) (-105.4142, 6.3044) (-105.0166, 6.3785) (-104.8214, 6.3785) knots 0 0 0 1 2 2 2
  spline S167 degree 2 poles (-104.8214, 6.3785) (-104.5843, 6.3785) (-104.2608, 6.3044) (-104.1323, 6.2081) knots 0 0 0 1 2 2 2
  spline S168 degree 2 poles (-104.1323, 6.2081) (-104.0063, 6.1142) (-103.8828, 5.8153) (-103.8828, 5.6004) knots 0 0 0 1 2 2 2
  line L135 (-103.8828, 5.6004) -> (-103.8828, 4.0369)
  line L136 (-103.8828, 4.0369) -> (-104.2682, 4.0369)
  line L137 (-104.2682, 4.0369) -> (-104.2682, 4.279)
  line L138 (-104.2682, 4.6001) -> (-104.2682, 5.2349)
  spline S169 degree 2 poles (-104.2682, 5.2349) (-104.4065, 5.2225) (-104.8239, 5.1805) (-104.9548, 5.141) knots 0 0 0 1 2 2 2
  spline S170 degree 2 poles (-104.9548, 5.141) (-105.108, 5.0941) (-105.308, 4.8989) (-105.308, 4.726) knots 0 0 0 1 2 2 2
  spline S171 degree 2 poles (-105.308, 4.726) (-105.308, 4.5284) (-105.0857, 4.3284) (-104.8733, 4.3284) knots 0 0 0 1 2 2 2
  spline S172 degree 2 poles (-104.8733, 4.3284) (-104.693, 4.3284) (-104.3966, 4.484) (-104.2682, 4.6001) knots 0 0 0 1 2 2 2
  line L139 (-102.9492, 4.0369) -> (-103.3345, 4.0369)
  line L140 (-103.3345, 4.0369) -> (-103.3345, 6.3241)
  line L141 (-103.3345, 6.3241) -> (-102.9492, 6.3241)
  line L142 (-102.9492, 6.3241) -> (-102.9492, 4.0369)
  line L143 (-102.922, 6.7045) -> (-103.3592, 6.7045)
  line L144 (-103.3592, 6.7045) -> (-103.3592, 7.1047)
  line L145 (-103.3592, 7.1047) -> (-102.922, 7.1047)
  line L146 (-102.922, 7.1047) -> (-102.922, 6.7045)
  point P0 (-5, 0)
  constraints: 2 other
extrude "Extrusion6" cut sketch "Sketch6" against normal blind 2
body "Solid1"
